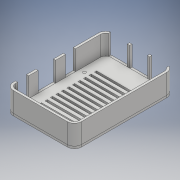
# Autodesk Inventor part: TapaChasisDron_P1
Saved by Autodesk Inventor 2017.3 (Build 213256000, 256)
## iProperties
Part Number: TapaChasisDron_P1
Material: Genérico
Document SubType Name: Modeling
Designer: danie
Density: 1 g/cm^3
Appearance: Valor por defecto
Author: danie
Autodesk Inventor part; units mm, degrees
ref_plane "YZ Plane" through (0, 0, 0) normal (1, 0, 0) x (0, 1, 0)
ref_plane "XZ Plane" through (0, 0, 0) normal (0, 1, 0) x (-1, 0, 0)
ref_plane "XY Plane" through (0, 0, 0) normal (0, 0, 1) x (1, 0, 0)
sketch "Boceto1" plane through (0, 0, 0) normal (0, 0, 1) x (1, 0, 0)
  line L0 (26.4667, -19.6479) -> (-22.5333, -19.6479) construction
  line L1 (-26.0333, -16.1479) -> (-26.0333, 61.1344) construction
  arc A0 (-26.0333, -16.1479) -> (-22.5333, -19.6479) centre (-22.5333, -16.1479) ccw construction
  arc A1 (26.4667, -19.6479) -> (29.9667, -16.1479) centre (26.4667, -16.1479) ccw construction
  arc A2 (29.9667, 61.1344) -> (26.4667, 64.6344) centre (26.4667, 61.1344) ccw construction
  arc A3 (-22.5333, 64.6344) -> (-26.0333, 61.1344) centre (-22.5333, 61.1344) ccw construction
  circle A4 centre (-22.5333, 41.8521) radius 1.375
  line L2 (-4.815, -3.944) -> (-4.815, 39.962) construction
  line L3 (-4.815, 39.962) -> (4.8805, 39.962) construction
  line L4 (4.8805, 39.962) -> (4.8805, -3.944) construction
  line L5 (4.8805, -3.944) -> (-4.815, -3.944) construction
  circle A5 centre (-22.5333, -16.1479) radius 1.375
  circle A6 centre (26.4667, -16.1479) radius 1.375
  line L6 (29.9667, 61.1344) -> (29.9667, -16.1479) construction
  line L7 (26.4667, 64.6344) -> (-22.5333, 64.6344) construction
  line L8 (-22.5333, -20.6479) -> (26.4667, -20.6479)
  arc A7 (26.4667, -20.6479) -> (30.9667, -16.1479) centre (26.4667, -16.1479) ccw
  line L9 (30.9667, -16.1479) -> (30.9667, 61.1344)
  arc A8 (30.9667, 61.1344) -> (26.4667, 65.6344) centre (26.4667, 61.1344) ccw
  line L10 (26.4667, 65.6344) -> (-22.5333, 65.6344)
  arc A9 (-22.5333, 65.6344) -> (-27.0333, 61.1344) centre (-22.5333, 61.1344) ccw
  line L11 (-27.0333, 61.1344) -> (-27.0333, -16.1479)
  arc A10 (-27.0333, -16.1479) -> (-22.5333, -20.6479) centre (-22.5333, -16.1479) ccw
  line L12 (26.4667, -22.6479) -> (-22.5333, -22.6479)
  arc A11 (-29.0333, -16.1479) -> (-22.5333, -22.6479) centre (-22.5333, -16.1479) ccw
  line L13 (-29.0333, -16.1479) -> (-29.0333, 61.1344)
  arc A12 (-22.5333, 67.6344) -> (-29.0333, 61.1344) centre (-22.5333, 61.1344) ccw
  line L14 (-22.5333, 67.6344) -> (26.4667, 67.6344)
  arc A13 (32.9667, 61.1344) -> (26.4667, 67.6344) centre (26.4667, 61.1344) ccw
  line L15 (32.9667, 61.1344) -> (32.9667, -16.1479)
  arc A14 (26.4667, -22.6479) -> (32.9667, -16.1479) centre (26.4667, -16.1479) ccw
  circle A15 centre (26.4667, 41.8521) radius 1.375
  line L16 (-25.0333, 64.6344) -> (-9.0333, 64.6344)
  line L17 (-9.0333, 64.6344) -> (-9.0333, 68.6344)
  line L18 (-9.0333, 68.6344) -> (-25.0333, 68.6344)
  line L19 (-25.0333, 68.6344) -> (-25.0333, 64.6344)
  line L20 (-25.0333, 64.6344) -> (-9.0333, 68.6344) construction
  line L21 (-9.0333, 64.6344) -> (-25.0333, 68.6344) construction
  circle A16 centre (-4.2556, 66.6344) radius 1 construction
  line L22 (-25.0333, 66.6344) -> (32.9515, 66.6344) construction
  line L23 (-7.0333, 64.6344) -> (8.9667, 64.6344)
  line L24 (8.9667, 64.6344) -> (8.9667, 68.6344)
  line L25 (8.9667, 68.6344) -> (-7.0333, 68.6344)
  line L26 (-7.0333, 68.6344) -> (-7.0333, 64.6344)
  line L27 (-7.0333, 64.6344) -> (8.9667, 68.6344) construction
  line L28 (8.9667, 64.6344) -> (-7.0333, 68.6344) construction
  line L29 (11.2167, 64.6344) -> (28.2167, 64.6344)
  line L30 (28.2167, 64.6344) -> (28.2167, 68.6344)
  line L31 (28.2167, 68.6344) -> (11.2167, 68.6344)
  line L32 (11.2167, 68.6344) -> (11.2167, 64.6344)
  line L33 (11.2167, 64.6344) -> (28.2167, 68.6344) construction
  line L34 (28.2167, 64.6344) -> (11.2167, 68.6344) construction
  circle A17 centre (-28.0333, 46.7254) radius 1 construction
  line L35 (-28.0333, 65.5936) -> (-28.0333, -17.0308) construction
  line L36 (-30.0333, 29.3521) -> (-26.0333, 29.3521)
  line L37 (-26.0333, 29.3521) -> (-26.0333, 38.3521)
  line L38 (-26.0333, 38.3521) -> (-30.0333, 38.3521)
  line L39 (-30.0333, 38.3521) -> (-30.0333, 29.3521)
  line L40 (-30.0333, 29.3521) -> (-26.0333, 38.3521) construction
  line L41 (-26.0333, 29.3521) -> (-30.0333, 38.3521) construction
  line L42 (-30.0333, 4.3521) -> (-26.0333, 4.3521)
  line L43 (-26.0333, 4.3521) -> (-26.0333, 20.3521)
  line L44 (-26.0333, 20.3521) -> (-30.0333, 20.3521)
  line L45 (-30.0333, 20.3521) -> (-30.0333, 4.3521)
  line L46 (-30.0333, 4.3521) -> (-26.0333, 20.3521) construction
  line L47 (-26.0333, 4.3521) -> (-30.0333, 20.3521) construction
  line L48 (-30.0333, -14.1479) -> (-26.0333, -14.1479)
  line L49 (-26.0333, -14.1479) -> (-26.0333, -4.1479)
  line L50 (-26.0333, -4.1479) -> (-30.0333, -4.1479)
  line L51 (-30.0333, -4.1479) -> (-30.0333, -14.1479)
  line L52 (-30.0333, -14.1479) -> (-26.0333, -4.1479) construction
  line L53 (-26.0333, -14.1479) -> (-30.0333, -4.1479) construction
  point P0 (0, 0)
  point P1 (0, 0)
  point P2 (29.9667, -19.6479)
  point P3 (-26.0333, -19.6479)
  point P4 (0, 0)
  point P5 (-17.0333, 66.6344)
  point P6 (-5.0179, 67.6344)
  point P7 (-5.0179, 65.6344)
  point P8 (-17.0333, 66.6344)
  point P9 (0.9667, 66.6344)
  point P10 (19.7167, 66.6344)
  point P11 (-28.0333, 33.8521)
  point P12 (-28.0333, 12.3521)
  point P13 (-28.0333, -9.1479)
  dimension "d0" = 56
  dimension "d4" = 2.75
  dimension "d6" = 58
  dimension "d25" = 2.75
  dimension "d26" = 2.75
  dimension "d51" = 1
  dimension "d52" = 2
  dimension "d53" = 49
  dimension "d54" = 3.5
  dimension "d55" = 3.5
  dimension "d56" = 2.75
  dimension "d57" = 16
  dimension "d58" = 4
  dimension "d60" = 47
  dimension "d61" = 3.5
  dimension "d62" = 3.5
  dimension "d63" = 16
  dimension "d64" = 4
  dimension "d65" = 29
  dimension "d66" = 17
  dimension "d67" = 4
  dimension "d68" = 10.25
  dimension "d69" = 9
  dimension "d70" = 4
  dimension "d71" = 16
  dimension "d72" = 4
  dimension "d73" = 10
  dimension "d74" = 10.5
  dimension "d75" = 32
  dimension "d76" = 53.5
  constraints: 100 end point, 24 point on circle, 18 centre point, 14 parallel, 14 point on line, 13 midpoint, 12 tangent, 6 horizontal, 6 perpendicular, 2 coincident, 2 equal radius, 2 vertical alignment, 1 horizontal alignment, 1 vertical, 16 other
  measures "d0" distance of point (29.967, -19.648) point (-26.033, -19.648)
  measures "d4" diameter of A4
  measures "d6" distance of A0.centre A4.centre
  measures "d25" diameter of A5
  measures "d26" diameter of A6
  measures "d51" distance between parallel lines of L0 L8
  measures "d52" distance between parallel lines of L8 L12
  measures "d53" distance of A1.centre A5.centre
  measures "d54" distance from line of L1 A0.centre
  measures "d55" distance of L0.end A0.centre
  measures "d56" diameter of A15
  measures "d57" distance of L18.end L17.end
  measures "d58" distance of L17.end L16.end
  measures "d60" distance from line of L6 point (-17.033, 66.634)
  measures "d61" distance of L0.start A1.centre
  measures "d62" distance from line of L6 A1.centre
  measures "d63" distance of L25.end L24.end
  measures "d64" distance of L24.end L23.end
  measures "d65" distance from line of L6 point (0.967, 66.634)
  measures "d66" distance of L31.end L30.end
  measures "d67" distance of L30.end L29.end
  measures "d68" distance from line of L6 point (19.717, 66.634)
  measures "d69" distance of L37.end L36.end
  measures "d70" distance of L44.end L43.end
  measures "d71" distance of L43.end L42.end
  measures "d72" distance of L50.end L49.end
  measures "d73" distance of L49.end L48.end
  measures "d74" distance from line of L0 point (-28.033, -9.148)
  measures "d75" distance from line of L0 point (-28.033, 12.352)
  measures "d76" distance from line of L0 point (-28.033, 33.852)
extrude "Extrusión7" add sketch "Boceto1" against normal blind 2 contours A10 L11 L48 L49 L50 L42 L43 L44 L36 L37 L38 A9 L19 L16 L17 L10 L26 L23 L24 L32 L29 L30 A8 L9 A7 L8 | L11 L50 L49 L48 | L30 L29 L32 L10 A8 | L11 L44 L43 L42 | L11 L38 L37 L36 | L24 L23 L26 L10 | L17 L16 L19 A9 L10
extrude "Extrusión8" add sketch "Boceto1" along normal blind 18 contours L8 A7 L9 A8 L30 A13 L15 A14 L12 A11 L13 L48 L11 A10 | L48 L13 L50 L11 | L50 L13 L42 L11 | A8 L10 L32 L14 A13 L30 | L42 L13 L44 L11 | L44 L13 L36 L11 | L10 L24 L14 L32 | L36 L13 L38 L11 | L10 L26 L14 L24 | L38 L13 A12 L19 A9 L11 | L10 L17 L14 L26 | L10 A9 L19 A12 L14 L17
extrude "Extrusión9" add sketch "Boceto1" against normal up to surface (2 mm away) separate body contours L8 A7 L9 A8 L30 A13 L15 A14 L12 A11 L13 L48 L11 A10 | L48 L13 L50 L11 | L50 L13 L42 L11 | A8 L10 L32 L14 A13 L30 | L42 L13 L44 L11 | L44 L13 L36 L11 | L10 L24 L14 L32 | L36 L13 L38 L11 | L10 L26 L14 L24 | L38 L13 A12 L19 A9 L11 | L10 L17 L14 L26 | L10 A9 L19 A12 L14 L17
sketch "Boceto5" plane through (0, 0, 18) normal (0, 0, 1) x (1, 0, 0)
  circle A0 centre (-22.5333, 41.8521) radius 1.375
  line L0 (-4.815, -3.944) -> (-4.815, 39.962) construction
  line L1 (4.8805, 39.962) -> (4.8805, -3.944) construction
  arc A1 (26.4667, -19.6479) -> (29.9667, -16.1479) centre (26.4667, -16.1479) ccw construction
  line L2 (26.4667, -19.6479) -> (-22.5333, -19.6479) construction
  line L3 (-26.0333, -16.1479) -> (-26.0333, 61.1344) construction
  line L4 (-4.815, 39.962) -> (4.8805, 39.962) construction
  arc A2 (-26.0333, -16.1479) -> (-22.5333, -19.6479) centre (-22.5333, -16.1479) ccw construction
  arc A3 (-22.5333, 64.6344) -> (-26.0333, 61.1344) centre (-22.5333, 61.1344) ccw construction
  line L5 (4.8805, -3.944) -> (-4.815, -3.944) construction
  arc A4 (29.9667, 61.1344) -> (26.4667, 64.6344) centre (26.4667, 61.1344) ccw construction
  circle A5 centre (-22.5333, -16.1479) radius 1.375
  circle A6 centre (26.4667, -16.1479) radius 1.375
  line L6 (29.9667, 61.1344) -> (29.9667, -16.1479) construction
  line L7 (26.4667, 64.6344) -> (-22.5333, 64.6344) construction
  line L8 (-22.5333, -20.6479) -> (26.4667, -20.6479)
  arc A7 (26.4667, -20.6479) -> (30.9667, -16.1479) centre (26.4667, -16.1479) ccw
  line L9 (30.9667, -16.1479) -> (30.9667, 61.1344)
  arc A8 (30.9667, 61.1344) -> (26.4667, 65.6344) centre (26.4667, 61.1344) ccw
  line L10 (26.4667, 65.6344) -> (-22.5333, 65.6344)
  arc A9 (-22.5333, 65.6344) -> (-27.0333, 61.1344) centre (-22.5333, 61.1344) ccw
  line L11 (-27.0333, 61.1344) -> (-27.0333, -16.1479)
  arc A10 (-27.0333, -16.1479) -> (-22.5333, -20.6479) centre (-22.5333, -16.1479) ccw
  line L12 (26.4667, -22.6479) -> (-22.5333, -22.6479)
  arc A11 (-29.0333, -16.1479) -> (-22.5333, -22.6479) centre (-22.5333, -16.1479) ccw
  line L13 (-29.0333, -16.1479) -> (-29.0333, 61.1344)
  arc A12 (-22.5333, 67.6344) -> (-29.0333, 61.1344) centre (-22.5333, 61.1344) ccw
  line L14 (-22.5333, 67.6344) -> (26.4667, 67.6344)
  arc A13 (32.9667, 61.1344) -> (26.4667, 67.6344) centre (26.4667, 61.1344) ccw
  line L15 (32.9667, 61.1344) -> (32.9667, -16.1479)
  arc A14 (26.4667, -22.6479) -> (32.9667, -16.1479) centre (26.4667, -16.1479) ccw
  circle A15 centre (24.125, 37.3929) radius 1.375
  circle A16 centre (-4.2556, 66.6344) radius 1 construction
  line L16 (-26.7903, 66.6344) -> (31.1945, 66.6344) construction
  circle A17 centre (-28.0333, 46.7254) radius 1 construction
  line L17 (-28.0333, 65.5936) -> (-28.0333, -17.0308) construction
  line L18 (-30.0333, 29.3521) -> (-26.0333, 29.3521)
  line L19 (-26.0333, 29.3521) -> (-26.0333, 38.3521)
  line L20 (-26.0333, 38.3521) -> (-30.0333, 38.3521)
  line L21 (-30.0333, 38.3521) -> (-30.0333, 29.3521)
  line L22 (-30.0333, 29.3521) -> (-26.0333, 38.3521) construction
  line L23 (-26.0333, 29.3521) -> (-30.0333, 38.3521) construction
  line L24 (-30.0333, 4.3521) -> (-26.0333, 4.3521)
  line L25 (-26.0333, 4.3521) -> (-26.0333, 20.3521)
  line L26 (-26.0333, 20.3521) -> (-30.0333, 20.3521)
  line L27 (-30.0333, 20.3521) -> (-30.0333, 4.3521)
  line L28 (-30.0333, 4.3521) -> (-26.0333, 20.3521) construction
  line L29 (-26.0333, 4.3521) -> (-30.0333, 20.3521) construction
  line L30 (-30.0333, -14.1479) -> (-26.0333, -14.1479)
  line L31 (-26.0333, -14.1479) -> (-26.0333, -4.1479)
  line L32 (-26.0333, -4.1479) -> (-30.0333, -4.1479)
  line L33 (-30.0333, -4.1479) -> (-30.0333, -14.1479)
  line L34 (-30.0333, -14.1479) -> (-26.0333, -4.1479) construction
  line L35 (-26.0333, -14.1479) -> (-30.0333, -4.1479) construction
  line L36 (-24.2833, 65.1344) -> (-7.2833, 65.1344)
  line L37 (-7.2833, 65.1344) -> (-7.2833, 68.1344)
  line L38 (-7.2833, 68.1344) -> (-24.2833, 68.1344)
  line L39 (-24.2833, 68.1344) -> (-24.2833, 65.1344)
  line L40 (-24.2833, 65.1344) -> (-7.2833, 68.1344) construction
  line L41 (-7.2833, 65.1344) -> (-24.2833, 68.1344) construction
  line L42 (-5.0333, 65.1344) -> (10.9667, 65.1344)
  line L43 (10.9667, 65.1344) -> (10.9667, 68.1344)
  line L44 (10.9667, 68.1344) -> (-5.0333, 68.1344)
  line L45 (-5.0333, 68.1344) -> (-5.0333, 65.1344)
  line L46 (-5.0333, 65.1344) -> (10.9667, 68.1344) construction
  line L47 (10.9667, 65.1344) -> (-5.0333, 68.1344) construction
  line L48 (12.9667, 64.6344) -> (28.9667, 64.6344)
  line L49 (28.9667, 64.6344) -> (28.9667, 68.6344)
  line L50 (28.9667, 68.6344) -> (12.9667, 68.6344)
  line L51 (12.9667, 68.6344) -> (12.9667, 64.6344)
  line L52 (12.9667, 64.6344) -> (28.9667, 68.6344) construction
  line L53 (28.9667, 64.6344) -> (12.9667, 68.6344) construction
  line L54 (-27.0333, -16.1479) -> (-27.0333, 61.1344) projected
  point P0 (0, 0)
  point P1 (0, 0)
  point P2 (29.9667, -19.6479)
  point P3 (-26.0333, -19.6479)
  point P4 (0, 0)
  point P5 (0, 0)
  point P6 (-5.0179, 65.6344)
  point P7 (-28.0333, 33.8521)
  point P8 (-28.0333, 12.3521)
  point P9 (-28.0333, -9.1479)
  point P10 (-15.7833, 66.6344)
  point P11 (2.9667, 66.6344)
  point P12 (20.9667, 66.6344)
  dimension "d83" = 56
  dimension "d84" = 2.75
  dimension "d85" = 58
  dimension "d86" = 2.75
  dimension "d87" = 2.75
  dimension "d88" = 1
  dimension "d89" = 2
  dimension "d90" = 49
  dimension "d91" = 3.5
  dimension "d92" = 3.5
  dimension "d93" = 2.75
  dimension "d97" = 3.5
  dimension "d98" = 3.5
  dimension "d105" = 9
  dimension "d106" = 4
  dimension "d107" = 16
  dimension "d108" = 4
  dimension "d109" = 10
  dimension "d110" = 10.5
  dimension "d111" = 32
  dimension "d112" = 53.5
  dimension "d147" = 17
  dimension "d148" = 3
  dimension "d149" = 16
  dimension "d150" = 3
  dimension "d151" = 16
  dimension "d152" = 4
  dimension "d153" = 10.25
  dimension "d154" = 29
  dimension "d155" = 47
  constraints: 100 end point, 24 point on circle, 18 centre point, 14 parallel, 13 point on line, 12 midpoint, 12 tangent, 6 horizontal, 6 perpendicular, 2 coincident, 2 equal radius, 1 collinear, 1 vertical, 1 vertical alignment, 16 other
  measures "d83" distance of point (29.967, -19.648) point (-26.033, -19.648)
  measures "d84" diameter of A0
  measures "d85" distance of A2.centre A0.centre
  measures "d86" diameter of A5
  measures "d87" diameter of A6
  measures "d88" distance between parallel lines of L2 L8
  measures "d89" distance between parallel lines of L8 L12
  measures "d90" distance of A1.centre A5.centre
  measures "d91" distance from line of L3 A2.centre
  measures "d92" distance of L2.end A2.centre
  measures "d93" diameter of A15
  measures "d97" distance of L2.start A1.centre
  measures "d98" distance from line of L6 A1.centre
  measures "d105" distance of L20.start L19.start
  measures "d106" distance of L26.end L25.end
  measures "d107" distance of L25.end L25.start
  measures "d108" distance of L33.start L31.end
  measures "d109" distance of L31.end L31.start
  measures "d110" distance from line of L2 point (-28.033, -9.148)
  measures "d111" distance from line of L2 point (-28.033, 12.352)
  measures "d112" distance from line of L2 point (-28.033, 33.852)
  measures "d147" distance of L38.end L37.end
  measures "d148" distance of L37.end L36.end
  measures "d149" distance of L44.end L43.end
  measures "d150" distance of L43.end L42.end
  measures "d151" distance of L50.end L49.end
  measures "d152" distance of L49.end L48.end
  measures "d153" distance from line of point (-15.783, 66.634) L3
  measures "d154" distance from line of L3 point (2.967, 66.634)
  measures "d155" distance from line of L3 point (20.967, 66.634)
extrude "Extrusión11" add sketch "Boceto1" against normal up to surface (2 mm away) separate body contours A4 | A5 | A6 | A15
sketch "Boceto6" plane through (0, 0, 0) normal (0, 0, 1) x (1, 0, 0)
  circle A0 centre (-22.5333, 41.8521) radius 1.375 projected
  circle A1 centre (-22.5333, -16.1479) radius 1.375 projected
  circle A2 centre (26.4667, -16.1479) radius 1.375 projected
  circle A3 centre (26.4667, 41.8521) radius 1.375 projected
  line L0 (-27.0333, 61.1344) -> (-27.0333, -16.1479) projected
  arc A4 (-27.0333, -16.1479) -> (-22.5333, -20.6479) centre (-22.5333, -16.1479) ccw projected
  line L1 (-22.5333, -20.6479) -> (26.4667, -20.6479) projected
  arc A5 (26.4667, -20.6479) -> (30.9667, -16.1479) centre (26.4667, -16.1479) ccw projected
  line L2 (30.9667, -16.1479) -> (30.9667, 61.1344) projected
  arc A6 (30.9667, 61.1344) -> (26.4667, 65.6344) centre (26.4667, 61.1344) ccw projected
  line L3 (26.4667, 65.6344) -> (-22.5333, 65.6344) projected
  arc A7 (-22.5333, 65.6344) -> (-27.0333, 61.1344) centre (-22.5333, 61.1344) ccw projected
  line L4 (-18.0333, 8.4932) -> (21.9667, 8.4932)
  line L5 (21.9667, 8.4932) -> (21.9667, 6.4932)
  line L6 (21.9667, 6.4932) -> (-18.0333, 6.4932)
  line L7 (-18.0333, 6.4932) -> (-18.0333, 8.4932)
  line L8 (-18.0333, 8.4932) -> (21.9667, 6.4932) construction
  line L9 (21.9667, 8.4932) -> (-18.0333, 6.4932) construction
  line L10 (-17.8583, 3.4932) -> (21.9667, 3.4932)
  line L11 (21.9667, 3.4932) -> (21.9667, 1.4932)
  line L12 (21.9667, 1.4932) -> (-17.8583, 1.4932)
  line L13 (-17.8583, 1.4932) -> (-17.8583, 3.4932)
  line L14 (-17.8583, 3.4932) -> (21.9667, 1.4932) construction
  line L15 (21.9667, 3.4932) -> (-17.8583, 1.4932) construction
  line L16 (-18.0513, 48.4932) -> (21.9487, 48.4932)
  line L17 (21.9487, 48.4932) -> (21.9487, 46.4932)
  line L18 (21.9487, 46.4932) -> (-18.0513, 46.4932)
  line L19 (-18.0513, 46.4932) -> (-18.0513, 48.4932)
  line L20 (-18.0513, 48.4932) -> (21.9487, 46.4932) construction
  line L21 (21.9487, 48.4932) -> (-18.0513, 46.4932) construction
  line L22 (-18.0513, 43.4932) -> (21.9487, 43.4932)
  line L23 (21.9487, 43.4932) -> (21.9487, 41.4932)
  line L24 (21.9487, 41.4932) -> (-18.0513, 41.4932)
  line L25 (-18.0513, 41.4932) -> (-18.0513, 43.4932)
  line L26 (-18.0513, 43.4932) -> (21.9487, 41.4932) construction
  line L27 (21.9487, 43.4932) -> (-18.0513, 41.4932) construction
  line L28 (-18.0513, 38.4932) -> (21.9487, 38.4932)
  line L29 (21.9487, 38.4932) -> (21.9487, 36.4932)
  line L30 (21.9487, 36.4932) -> (-18.0513, 36.4932)
  line L31 (-18.0513, 36.4932) -> (-18.0513, 38.4932)
  line L32 (-18.0513, 38.4932) -> (21.9487, 36.4932) construction
  line L33 (21.9487, 38.4932) -> (-18.0513, 36.4932) construction
  line L34 (-18.0513, 33.4932) -> (21.9487, 33.4932)
  line L35 (21.9487, 33.4932) -> (21.9487, 31.4932)
  line L36 (21.9487, 31.4932) -> (-18.0513, 31.4932)
  line L37 (-18.0513, 31.4932) -> (-18.0513, 33.4932)
  line L38 (-18.0513, 33.4932) -> (21.9487, 31.4932) construction
  line L39 (21.9487, 33.4932) -> (-18.0513, 31.4932) construction
  line L40 (-18.0513, 28.4932) -> (21.9487, 28.4932)
  line L41 (21.9487, 28.4932) -> (21.9487, 26.4932)
  line L42 (21.9487, 26.4932) -> (-18.0513, 26.4932)
  line L43 (-18.0513, 26.4932) -> (-18.0513, 28.4932)
  line L44 (-18.0513, 28.4932) -> (21.9487, 26.4932) construction
  line L45 (21.9487, 28.4932) -> (-18.0513, 26.4932) construction
  line L46 (-18.0153, 23.4932) -> (21.9487, 23.4932)
  line L47 (21.9487, 23.4932) -> (21.9487, 21.4932)
  line L48 (21.9487, 21.4932) -> (-18.0153, 21.4932)
  line L49 (-18.0153, 21.4932) -> (-18.0153, 23.4932)
  line L50 (-18.0153, 23.4932) -> (21.9487, 21.4932) construction
  line L51 (21.9487, 23.4932) -> (-18.0153, 21.4932) construction
  line L52 (-18.0333, 18.4932) -> (21.9667, 18.4932)
  line L53 (21.9667, 18.4932) -> (21.9667, 16.4932)
  line L54 (21.9667, 16.4932) -> (-18.0333, 16.4932)
  line L55 (-18.0333, 16.4932) -> (-18.0333, 18.4932)
  line L56 (-18.0333, 18.4932) -> (21.9667, 16.4932) construction
  line L57 (21.9667, 18.4932) -> (-18.0333, 16.4932) construction
  line L58 (-18.0333, 13.4932) -> (21.9667, 13.4932)
  line L59 (21.9667, 13.4932) -> (21.9667, 11.4932)
  line L60 (21.9667, 11.4932) -> (-18.0333, 11.4932)
  line L61 (-18.0333, 11.4932) -> (-18.0333, 13.4932)
  line L62 (-18.0333, 13.4932) -> (21.9667, 11.4932) construction
  line L63 (21.9667, 13.4932) -> (-18.0333, 11.4932) construction
  circle A8 centre (1.9667, 65.9715) radius 29 construction
  line L64 (30.9667, 61.1344) -> (30.9667, -16.1479) projected
  line L65 (-27.0333, -16.1479) -> (-27.0333, 61.1344) projected
  line L66 (1.9667, 65.9715) -> (1.9667, -35.5731) construction
  circle A9 centre (1.9667, 22.4932) radius 43.1412 construction
  line L67 (26.4667, 65.6344) -> (-22.5333, 65.6344) projected
  line L68 (26.4667, -20.6479) -> (-22.5333, -20.6479) projected
  line L69 (-18.0333, -1.5068) -> (21.9667, -1.5068)
  line L70 (21.9667, -1.5068) -> (21.9667, -3.5068)
  line L71 (21.9667, -3.5068) -> (-18.0333, -3.5068)
  line L72 (-18.0333, -3.5068) -> (-18.0333, -1.5068)
  line L73 (-18.0333, -1.5068) -> (21.9667, -3.5068) construction
  line L74 (21.9667, -1.5068) -> (-18.0333, -3.5068) construction
  line L75 (1.9667, 22.4932) -> (35.1577, 22.4932)
  point P0 (0, 0)
  point P1 (8.9667, 65.6344)
  point P2 (-7.0333, 65.6344)
  point P3 (-27.0333, 38.3521)
  point P4 (1.9667, 7.4932)
  point P5 (2.0542, 2.4932)
  point P6 (1.9487, 47.4932)
  point P7 (1.9487, 42.4932)
  point P8 (1.9487, 37.4932)
  point P9 (1.9487, 32.4932)
  point P10 (1.9487, 27.4932)
  point P11 (1.9667, 22.4932)
  point P12 (1.9667, 17.4932)
  point P13 (1.9667, 12.4932)
  point P14 (1.9487, 47.4932)
  point P15 (1.9487, 42.4932)
  point P16 (1.9487, 37.4932)
  point P17 (1.9487, 32.4932)
  point P18 (1.9487, 27.4932)
  point P19 (1.9487, 32.4932)
  point P20 (1.9667, 17.4932)
  point P21 (1.9667, 22.4932)
  point P22 (1.9667, 7.4932)
  point P23 (1.9667, 12.4932)
  point P24 (1.9487, 42.4932)
  point P25 (1.9487, 37.4932)
  point P26 (1.9667, 22.4932)
  point P27 (1, 1)
  point P28 (1.9667, -2.5068)
  point P29 (1.9667, -2.5068)
  dimension "d117" = 40
  dimension "d118" = 2
  dimension "d119" = 2
  dimension "d120" = 3
  dimension "d121" = 40
  dimension "d122" = 2
  dimension "d123" = 2
  dimension "d124" = 3
  dimension "d125" = 40
  dimension "d126" = 2
  dimension "d127" = 2
  dimension "d128" = 3
  dimension "d129" = 40
  dimension "d130" = 2
  dimension "d131" = 2
  dimension "d132" = 3
  dimension "d133" = 40
  dimension "d134" = 2
  dimension "d135" = 2
  dimension "d136" = 3
  dimension "d137" = 3
  dimension "d138" = 3
  dimension "d139" = 3
  dimension "d140" = 3
  dimension "d141" = 2
  dimension "d142" = 3
  constraints: 136 end point, 36 midpoint, 22 parallel, 12 horizontal, 11 perpendicular, 8 point on line, 6 vertical alignment, 4 tangent, 2 centre point, 1 coincident, 1 vertical
  measures "d117" distance of L5.end L6.end
  measures "d118" distance of L4.end L5.end
  measures "d119" distance of L10.end L11.end
  measures "d120" distance between parallel lines of L10 L6
  measures "d121" distance of L18.start L18.end
  measures "d122" distance of L16.end L18.start
  measures "d123" distance of L22.end L23.end
  measures "d124" distance between parallel lines of L22 L18
  measures "d125" distance of L30.start L30.end
  measures "d126" distance of L28.end L30.start
  measures "d127" distance of L34.end L35.end
  measures "d128" distance between parallel lines of L34 L30
  measures "d129" distance of L42.start L42.end
  measures "d130" distance of L40.end L42.start
  measures "d131" distance of L46.end L47.end
  measures "d132" distance between parallel lines of L46 L42
  measures "d133" distance of L54.start L54.end
  measures "d134" distance of L52.end L54.start
  measures "d135" distance of L58.end L59.end
  measures "d136" distance between parallel lines of L58 L54
  measures "d137" distance between parallel lines of L28 L24
  measures "d138" distance between parallel lines of L40 L36
  measures "d139" distance between parallel lines of L52 L48
  measures "d140" distance between parallel lines of L4 L60
  measures "d141" distance of L69.end L70.end
  measures "d142" distance between parallel lines of L69 L12
extrude "Extrusión12" cut sketch "Boceto6" against normal through all contours L47 L48 L49 L46 | L4 L5 L6 L7 | L10 L11 L12 L13 | L16 L17 L18 L19 | L22 L23 L24 L25 | L28 L29 L30 L31 | L34 L35 L36 L37 | L40 L41 L42 L43 | L52 L53 L54 L55 | L58 L59 L60 L61 | L69 L70 L71 L72 bodies 1
extrude "Extrusión13" cut sketch "Boceto5" against normal up to surface (18 mm away) contours L30 L13 L32 L11 | L11 L32 L31 L30 | L30 L33 L32 L13 | L49 L48 L51 L10 A8 | A8 L10 L51 L14 A13 L49 | L24 L13 L26 L11 | L11 L26 L25 L24 | A13 L14 L51 L50 L49 | L24 L27 L26 L13 | L18 L13 L20 L11 | L11 L20 L19 L18 | L43 L42 L45 L10 | L10 L45 L14 L43 | L18 L21 L20 L13 | L14 L45 L44 L43 | L37 L36 L39 A9 L10 | L10 A9 L39 A12 L14 L37 | L14 A12 L39 L38 L37 bodies 1
equation "\"d64\" = d58"
equation "\"d67\" = d58"
